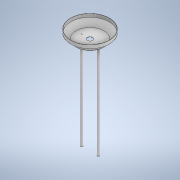
# Autodesk Inventor part: base
Saved by Autodesk Inventor 2021 (Build 250183000, 183)
## iProperties
Created: 2021-10-26
Part Number: base
Material: Genérico
Document SubType Name: Modeling
Designer: arthu
Density: 1 g/cm^3
Appearance: Valor por defecto
Author: arthu
Autodesk Inventor part; units mm, degrees
ref_plane "YZ Plane" through (0, 0, 0) normal (1, 0, 0) x (0, 1, 0)
ref_plane "XZ Plane" through (0, 0, 0) normal (0, 1, 0) x (-1, 0, 0)
ref_plane "XY Plane" through (0, 0, 0) normal (0, 0, 1) x (1, 0, 0)
sketch "Boceto1" plane through (0, 0, 0) normal (0, 1, 0) x (-1, 0, 0)
  circle A0 centre (0, 0) radius 90
  dimension "d0" = 180
  constraints: 1 centre point, 1 coincident
  measures "d0" diameter of A0
extrude "Extrusión1" add sketch "Boceto1" along normal blind 15
extrude "Extrusión2" add sketch "Boceto1" against normal blind 25 draft -45
shell "Vaciado1" thickness 1 removed faces 1 at (19.6237, 15, 24.7178)
sketch "Boceto2" plane through (0, -25, 0) normal (0, -1, 0) x (1, 0, 0)
  circle A0 centre (0, 0) radius 12.5
  dimension "d6" = 25
  constraints: 1 centre point, 1 coincident
  measures "d6" diameter of A0
extrude "Extrusión3" cut sketch "Boceto2" against normal blind 25
sketch "Boceto3" plane through (0, -25, 0) normal (0, -1, 0) x (1, 0, 0)
  circle A0 centre (0, 0) radius 12.5 projected
  circle A1 centre (0, 0) radius 45
  circle A2 centre (0, 0) radius 44
  line L0 (44, 0) -> (41.5, 0)
  circle A3 centre (41.5, 0) radius 2.5
  line L1 (-44, 0) -> (-41.5, 0)
  circle A4 centre (-41.5, 0) radius 2.5
  circle A5 centre (0, 41.5) radius 2.5
  circle A6 centre (-41.5, 0) radius 2.5
  circle A7 centre (0, -41.5) radius 2.5
  line L2 (44, 0) -> (39, 0)
  circle A8 centre (39, 0) radius 5
  circle A9 centre (-39, 0) radius 5
  point P0 (0, 44)
  point P1 (-44, 0)
  point P2 (0, -44)
  dimension "d9" = 90
  dimension "d10" = 88
  dimension "d11" = 2.5
  dimension "d12" = 2.5
  dimension "d13" = 5
  dimension "d16" = 360
  constraints: 6 end point, 6 point on circle, 5 centre point, 5 coincident, 3 horizontal, 2 horizontal alignment, 2 vertical alignment, 21 other
  measures "d9" diameter of A1
  measures "d10" diameter of A2
  measures "d11" distance of L0.start L0.end
  measures "d12" distance of L1.start L1.end
  measures "d13" diameter of A4
extrude "Extrusión4" add sketch "Boceto3" along normal blind 450 contours A4 | A9 | A3 L2 L0 | L0 L2 A3 | A8
shell "Vaciado2" thickness 1 removed faces 2 at (-39.591, -475, 0.7606) at (39.8768, -475, -0.3989)
